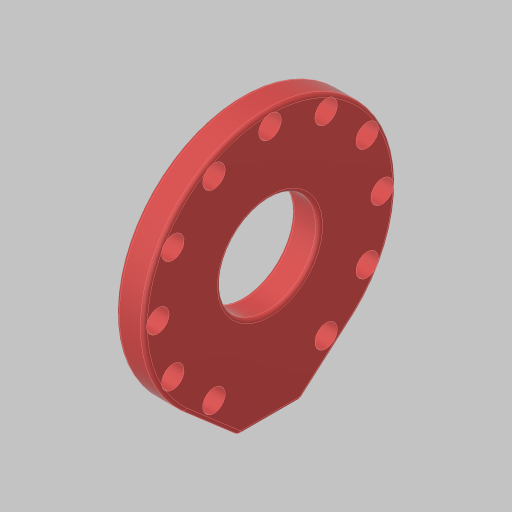
# Autodesk Inventor part: X 60 MOTOR SPACER
Saved by Autodesk Inventor 2023.5 (Build 275446000, 446)
## iProperties
Created: 2025-03-09
Part Number: X 60 MOTOR SPACER
Material: ABS Plastic
Document SubType Name: Modeling
Designer: slick
Density: 1.06 g/cm^3
Appearance: Smooth - Red
Author: slick
Autodesk Inventor part; units mm, degrees
ref_plane "YZ Plane" through (0, 0, 0) normal (1, 0, 0) x (0, 1, 0)
ref_plane "XZ Plane" through (0, 0, 0) normal (0, 1, 0) x (-1, 0, 0)
ref_plane "XY Plane" through (0, 0, 0) normal (0, 0, 1) x (1, 0, 0)
sketch "Sketch1" plane through (0, 0, 0) normal (1, 0, 0) x (0, 1, 0)
  circle A0 centre (0, 0) radius 28.575
  line L0 (-31.75, 6.985) -> (-31.75, -6.985)
  line L1 (-31.75, 6.985) -> (-21.0157, 19.3615)
  line L2 (-31.75, -6.985) -> (-21.0157, -19.3615)
  circle A1 centre (0, 0) radius 25.4 construction
  circle A2 centre (0, 0) radius 11.1125
  point P0 (25.4, 0)
  point P1 (21.997, 12.7)
  point P2 (12.7, 21.997)
  point P3 (0, 25.4)
  point P4 (-12.7, 21.997)
  point P5 (-21.997, 12.7)
  point P6 (-25.4, 0)
  point P7 (-21.997, -12.7)
  point P8 (-12.7, -21.997)
  point P9 (0, -25.4)
  point P10 (12.7, -21.997)
  point P11 (21.997, -12.7)
  dimension "d7" = 50.8
  dimension "d0" = 57.15
  dimension "d1" = 31.75
  dimension "d4" = 16.383
  dimension "d5" = 13.97
  dimension "d10" = 360
  dimension "d22" = 22.225
  constraints: 6 end point, 3 coincident, 2 centre point, 2 horizontal alignment, 2 point on circle, 1 equal length, 1 vertical, 1 vertical alignment, 15 other
  measures "d0" diameter of A0
  measures "d1" distance from line of point (0, 0) L0
  measures "d4" distance of L2.end L0.end
  measures "d5" distance of L0.start L0.end
  measures "d22" diameter of A2
extrude "Extrusion1" add sketch "Sketch1" along normal blind 6.35 contours A0 L2 L1 | A0 L2 L0 L1
hole "Hole1" at (0, 25.4, 0) at (0, 21.997, 12.7) at (0, 12.7, 21.997) at (0, 0, 25.4) at (0, -12.7, 21.997) at (0, -21.997, 12.7) at (0, -21.997, -12.7) at (0, -12.7, -21.997) at (0, 0, -25.4) at (0, 12.7, -21.997) at (0, 21.997, -12.7) direction (1, 0, 0) diameter 5.1054 end through all clearance for "Flat Head Machine Screw (82)" size "#10" standard "Ansi Unified Screw Threads"
fillet "Fillet1" radius 0.7937 12 edges at (6.35, 28.575, 0) (0, 28.575, 0) (6.35, -26.3829, 13.1733) (0, -26.3829, 13.1733) (6.35, -31.75, 0) (6.35, -26.3829, -13.1733) (0, -26.3829, -13.1733) (0, -31.75, 0) (3.175, -31.75, -6.985) (3.175, -31.75, 6.985) (0, -11.1125, 0) (6.35, -11.1125, 0)
body "Solid1"
